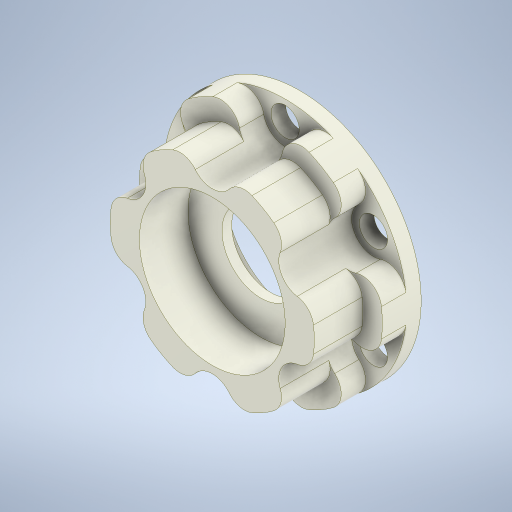
# Autodesk Inventor part: motor_top
Saved by Autodesk Inventor 2023.1 (Build 271208000, 208)
## iProperties
Created: 2019-06-25
Part Number: motor_top
Material: Polytetrafluoroethylene
Document SubType Name: Modeling
Designer: Timo
Density: 2.02 g/cm^3
Appearance: Smooth - Ivory
Author: Timo
Autodesk Inventor part; units mm, degrees
ref_plane "YZ Plane" through (0, 0, 0) normal (1, 0, 0) x (0, 1, 0)
ref_plane "XZ Plane" through (0, 0, 0) normal (0, 1, 0) x (-1, 0, 0)
ref_plane "XY Plane" through (0, 0, 0) normal (0, 0, 1) x (1, 0, 0)
sketch "Sketch1" plane through (0, 0, 0) normal (0, 0, 1) x (1, 0, 0)
  circle A0 centre (0, 0) radius 12.5
  dimension "d0" = 25
  constraints: 1 centre point, 1 coincident
  measures "d0" diameter of A0
extrude "Extrusion1" add sketch "Sketch1" along normal blind 9.5
sketch "Sketch2" plane through (0, 0, 9.5) normal (0, 0, 1) x (1, 0, 0)
  line L0 (0, 17.5) -> (0, -17.5) projected
  point P0 (0, 0)
  point P1 (0, 10.5)
  point P2 (-9.0933, 5.25)
  point P3 (-9.0933, -5.25)
  point P4 (0, -10.5)
  point P5 (9.0933, -5.25)
  point P6 (9.0933, 5.25)
  dimension "d3" = 10.5
  dimension "d6" = 360
  constraints: 1 point on line, 7 other
  measures "d3" distance of point (0, 0) point (0, 10.5)
hole "Hole1" at (0, 10.5, 9.5) at (-9.0933, 5.25, 9.5) at (-9.0933, -5.25, 9.5) at (0, -10.5, 9.5) at (9.0933, 5.25, 9.5) at (9.0933, -5.25, 9.5) direction (0, 0, -1) diameter 2.9 depth 9.5 counterbore diameter 4.5 counterbore depth 8 clearance for "Socket Head Cap Screw" size "M2.5" standard "Ansi Metric M Profile"
sketch "Sketch3" plane through (0, 0, 0) normal (0, 0, -1) x (-1, 0, 0)
  circle A0 centre (0, 0) radius 7.75
  dimension "d15" = 15.5
  constraints: 1 centre point, 1 coincident
  measures "d15" diameter of A0
extrude "Extrusion2" cut sketch "Sketch3" against normal blind 3
sketch "Sketch4" plane through (0, 0, 9.5) normal (0, 0, 1) x (1, 0, 0)
  circle A0 centre (0, 0) radius 7.5
  dimension "d18" = 15
  constraints: 1 centre point, 1 coincident
  measures "d18" diameter of A0
extrude "Extrusion3" cut sketch "Sketch4" against normal blind 5.5
sketch "Sketch5" plane through (0, 0, 9.5) normal (0, 0, 1) x (1, 0, 0)
  circle A0 centre (0, 10.5) radius 1.45 projected
  circle A1 centre (0, 0) radius 10.5
  circle A2 centre (0, 0) radius 12.5
  point P0 (-1.4465, 10.3999)
  point P1 (1.4465, 10.3999)
  constraints: 2 coincident, 1 centre point, 3 other
extrude "Extrusion4" cut sketch "Sketch5" against normal blind 5.5
sketch "Sketch6" plane through (0, 0, 4) normal (0, 0, 1) x (1, 0, 0)
  circle A0 centre (0, 0) radius 4
  dimension "d23" = 8
  constraints: 1 centre point, 1 coincident
  measures "d23" diameter of A0
extrude "Extrusion5" cut sketch "Sketch6" against normal through all
fillet "Fillet1" radius 2 4 edges at (1.1235, -12.4494, 2.75) (-1.1235, -12.4494, 2.75) (2.237, -10.2589, 6.75) (-2.237, -10.2589, 6.75)
pattern_circular "Circular Pattern1" count 6 over 360 about axis through (0, 0, -10) along (0, 0, 1) of "Fillet1"
sketch "Sketch7" plane through (0, 0, 9.5) normal (0, 0, 1) x (1, 0, 0)
  circle A0 centre (0, 0) radius 17.1567
  constraints: 1 centre point, 1 coincident
extrude "Extrusion6" cut sketch "Sketch7" against normal blind 0.5
body "Solid1"
